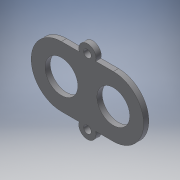
# Autodesk Inventor part: Inverter Housing Half 2
Saved by Autodesk Inventor 2019.4 (Build 234330000, 330)
## iProperties
Created: 2020-02-16
Part Number: Inverter Housing Half 2
Material: Generic
Document SubType Name: Modeling
Designer: admin
Density: 1 g/cm^3
Appearance: Default
Author: admin
Autodesk Inventor part; units mm, degrees
ref_plane "YZ Plane" through (0, 0, 0) normal (1, 0, 0) x (0, 1, 0)
ref_plane "XZ Plane" through (0, 0, 0) normal (0, 1, 0) x (-1, 0, 0)
ref_plane "XY Plane" through (0, 0, 0) normal (0, 0, 1) x (1, 0, 0)
sketch "Sketch1" plane through (0, 0, 0) normal (0, 0, 1) x (1, 0, 0)
  circle A0 centre (-15, 0) radius 9.5
  circle A1 centre (15, 0) radius 9.5
  line L0 (15, 0) -> (-15, 0) construction
  line L1 (-15, 0) -> (15, 0) construction
  line L2 (-15, -17.5) -> (-4.7727, -17.5)
  line L3 (15, 17.5) -> (4.7727, 17.5)
  arc A2 (-15, 17.5) -> (-15, -17.5) centre (-15, 0) ccw
  arc A3 (15, -17.5) -> (15, 17.5) centre (15, 0) ccw
  circle A4 centre (0, -18.9905) radius 2.2 projected
  circle A5 centre (0, 18.9905) radius 2.2 projected
  arc A6 (-4.7727, -17.5) -> (4.7727, -17.5) centre (0, -18.9905) ccw
  arc A7 (4.7727, 17.5) -> (-4.7727, 17.5) centre (0, 18.9905) ccw
  arc A8 (4.7727, -17.5) -> (-4.7727, -17.5) centre (0, -18.9905) ccw construction
  line L4 (-1.6181, -17.5) -> (1.6181, -17.5) construction
  line L5 (1.6181, -17.5) -> (4.7727, -17.5) construction
  line L6 (-4.7727, -17.5) -> (-1.6181, -17.5) construction
  line L7 (4.7727, -17.5) -> (15, -17.5)
  arc A9 (-4.7727, 17.5) -> (4.7727, 17.5) centre (0, 18.9905) ccw construction
  line L8 (-1.6181, 17.5) -> (-4.7727, 17.5) construction
  line L9 (-4.7727, 17.5) -> (-15, 17.5)
  line L10 (1.6181, 17.5) -> (-1.6181, 17.5) construction
  line L11 (4.7727, 17.5) -> (1.6181, 17.5) construction
  point P0 (0, 0)
  point P1 (0, 0)
  point P2 (0, 0)
  dimension "d0" = 19
  dimension "d1" = 19
  dimension "d2" = 30
  dimension "d3" = 35
  dimension "d6" = 10
  dimension "d7" = 10
  constraints: 26 end point, 25 parallel, 20 tangent, 16 point on circle, 8 centre point, 3 coincident, 3 point on line, 2 midpoint, 1 collinear, 1 horizontal
  measures "d0" diameter of A0
  measures "d1" diameter of A1
  measures "d2" distance of L0.end L0.start
  measures "d3" diameter of A3
  measures "d6" diameter of A6
  measures "d7" diameter of A7
extrude "Extrusion1" add sketch "Sketch1" along normal blind 3
fillet "Fillet1" radius 10 4 edges at (-4.7727, -17.5, 1.5) (4.7727, -17.5, 1.5) (-4.7727, 17.5, 1.5) (4.7727, 17.5, 1.5)
body "Solid1"
